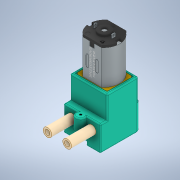
# Autodesk Inventor part: MPP20-E20
Saved by Autodesk Inventor 2020.4 (Build 244396010, 396A)
## iProperties
Created: 2021-10-01
Part Number: MPP20-E20
Material: Generic
Document SubType Name: Modeling
Designer: jonathanlim
Density: 1 g/cm^3
Appearance: Default
Author: jonathanlim
Autodesk Inventor part; units mm, degrees
ref_plane "YZ Plane" through (0, 0, 0) normal (1, 0, 0) x (0, 1, 0)
ref_plane "XZ Plane" through (0, 0, 0) normal (0, 1, 0) x (-1, 0, 0)
ref_plane "XY Plane" through (0, 0, 0) normal (0, 0, 1) x (1, 0, 0)
sketch "Sketch1" plane through (0, 0, 0) normal (0, 1, 0) x (-1, 0, 0)
  line L0 (-7.5, 8.3) -> (7.5, 8.3)
  line L1 (7.5, 8.3) -> (7.5, -8.3)
  line L2 (7.5, -8.3) -> (-7.5, -8.3)
  line L3 (-7.5, -8.3) -> (-7.5, 8.3)
  line L4 (-7.5, 8.3) -> (7.5, -8.3) construction
  line L5 (7.5, 8.3) -> (-7.5, -8.3) construction
  point P0 (0, 0)
  dimension "d0" = 15
  dimension "d1" = 16.6
  constraints: 12 end point, 2 midpoint, 2 parallel, 1 horizontal, 1 perpendicular
  measures "d0" distance of L1.end L2.end
  measures "d1" distance of L0.end L1.end
extrude "Extrusion1" add sketch "Sketch1" along normal blind 10.35
sketch "Sketch2" plane through (0, 10.35, 0) normal (0, 1, 0) x (1, 0, 0)
  line L0 (-7.5, -5.55) -> (7.5, -5.55)
  line L1 (7.5, -5.55) -> (7.5, 7.25)
  line L2 (7.5, 7.25) -> (-7.5, 7.25)
  line L3 (-7.5, 7.25) -> (-7.5, -5.55)
  line L4 (-7.5, -5.55) -> (7.5, 7.25) construction
  line L5 (7.5, -5.55) -> (-7.5, 7.25) construction
  line L6 (-7.5, -8.3) -> (7.5, -8.3) projected
  point P0 (0, 0)
  point P1 (0, 0.85)
  point P2 (0, 0.85)
  dimension "d4" = 12.8
  dimension "d5" = 2.75
  constraints: 12 end point, 3 midpoint, 2 parallel, 1 horizontal, 1 perpendicular, 1 vertical alignment
  measures "d4" distance of L1.end L0.end
  measures "d5" distance between parallel lines of L6 L0
extrude "Extrusion2" add sketch "Sketch2" along normal blind 9.2
sketch "Sketch3" plane through (0, 19.55, 0) normal (0, 1, 0) x (1, 0, 0)
  line L0 (-3.8, -4.15) -> (3.8, -4.15)
  line L1 (3.8, -4.15) -> (3.8, 5.85)
  line L2 (3.8, 5.85) -> (-3.8, 5.85)
  line L3 (-3.8, 5.85) -> (-3.8, -4.15)
  line L4 (-3.8, -4.15) -> (3.8, 5.85) construction
  line L5 (3.8, -4.15) -> (-3.8, 5.85) construction
  line L6 (-7.5, 7.25) -> (-7.5, -5.55)
  line L7 (7.5, 7.25) -> (-7.5, 7.25)
  arc A0 (-3.8, 5.85) -> (-3.8, -4.15) centre (0.353312, 0.85) ccw
  arc A1 (3.8, -4.15) -> (3.8, 5.85) centre (-0.353312, 0.85) ccw
  point P0 (0, 0.85)
  dimension "d10" = 7.6
  dimension "d11" = 10
  dimension "d12" = 7.5
  dimension "d13" = 1.4
  dimension "d14" = 6.5
  constraints: 12 end point, 4 point on circle, 2 centre point, 2 midpoint, 2 parallel, 1 equal radius, 1 horizontal, 1 perpendicular
  measures "d10" distance of L2.end L1.end
  measures "d11" distance of L1.end L0.end
  measures "d12" distance from line of L6 point (0, 0.85)
  measures "d13" distance between parallel lines of L7 L2
  measures "d14" radius of A0
extrude "Extrusion3" add sketch "Sketch3" along normal blind 14 separate body
sketch "Sketch6" plane through (0, 10.35, 0) normal (0, 1, 0) x (1, 0, 0)
  arc A0 (-1.910661, -8.3) -> (1.910661, -8.3) centre (0, -8.8) ccw
  line L0 (-7.5, -8.3) -> (7.5, -8.3)
  line L1 (-7.5, -8.3) -> (7.5, -8.3)
  line L2 (-1.910661, -8.3) -> (1.910661, -8.3)
  point P0 (0, 0)
  point P1 (1.910661, -8.3)
  point P2 (-1.910661, -8.3)
  dimension "d24" = 3.95
  dimension "d25" = 0.5
  constraints: 2 end point, 2 point on circle, 2 point on line, 1 centre point
  measures "d24" diameter of A0
  measures "d25" distance from line of L0 A0.centre
extrude "Extrusion6" add sketch "Sketch6" against normal blind 5.55 bodies 1
sketch "Sketch7" plane through (0, 0, 0) normal (0, -1, 0) x (1, 0, 0)
  circle A0 centre (0, 8.8) radius 1.975
  line L0 (-7.5, 8.3) -> (7.5, 8.3) projected
  point P0 (0, 0)
  dimension "d28" = 3.95
  dimension "d29" = 0.5
  constraints: 1 centre point
  measures "d28" diameter of A0
  measures "d29" distance from line of L0 A0.centre
extrude "Extrusion7" cut sketch "Sketch7" against normal up to surface (4.8 mm away) bodies 1
sketch "Sketch8" plane through (7.5, 0, 8.3) normal (0, 0, 1) x (1, 0, 0)
  circle A0 centre (-3.5, 6.85) radius 1.75
  circle A1 centre (-11.5, 6.85) radius 1.75
  line L0 (0, 0) -> (0, 10.35)
  line L1 (-5.589339, 10.35) -> (0, 10.35)
  point P0 (-7.5, 0)
  dimension "d32" = 3.5
  dimension "d33" = 8
  dimension "d34" = 3.5
  dimension "d37" = 3.5
  constraints: 2 centre point, 1 equal radius, 1 horizontal alignment
  measures "d32" diameter of A0
  measures "d33" distance of A0.centre A1.centre
  measures "d34" distance from line of L0 A0.centre
  measures "d37" distance from line of L1 A0.centre
extrude "Extrusion8" add sketch "Sketch8" along normal blind 10 separate body
sketch "Sketch12" plane through (0, 19.55, 0) normal (0, 1, 0) x (1, 0, 0)
  line L0 (-5.35, -4.4) -> (5.35, -4.4)
  line L1 (6.35, -3.4) -> (6.35, 5.1)
  line L2 (5.35, 6.1) -> (-5.35, 6.1)
  line L3 (-6.35, 5.1) -> (-6.35, -3.4)
  line L4 (-6.35, -4.4) -> (6.35, 6.1) construction
  line L5 (6.35, -4.4) -> (-6.35, 6.1) construction
  line L6 (7.5, -5.55) -> (7.5, 7.25) projected
  line L7 (7.5, 7.25) -> (-7.5, 7.25) projected
  line L8 (-7.5, -5.55) -> (7.5, -5.55) projected
  line L9 (-7.5, 7.25) -> (-7.5, -5.55) projected
  arc A0 (-5.35, 6.1) -> (-6.35, 5.1) centre (-5.35, 5.1) ccw
  arc A1 (6.35, 5.1) -> (5.35, 6.1) centre (5.35, 5.1) ccw
  arc A2 (5.35, -4.4) -> (6.35, -3.4) centre (5.35, -3.4) ccw
  arc A3 (-6.35, -3.4) -> (-5.35, -4.4) centre (-5.35, -3.4) ccw
  line L10 (-6.5, -4.55) -> (6.5, -4.55)
  line L11 (6.5, -4.55) -> (6.5, 6.25)
  line L12 (6.5, 6.25) -> (-6.5, 6.25)
  line L13 (-6.5, 6.25) -> (-6.5, -4.55)
  line L14 (-6.5, -4.55) -> (6.5, 6.25) construction
  line L15 (6.5, -4.55) -> (-6.5, 6.25) construction
  point P0 (0, 0)
  point P1 (0, 0.85)
  dimension "d52" = 1.15
  dimension "d53" = 1.15
  dimension "d54" = 1.15
  dimension "d55" = 1.15
  dimension "d56" = 1
  dimension "d57" = 1
  dimension "d58" = 1
  constraints: 24 end point, 8 point on circle, 8 point on line, 8 tangent, 4 centre point, 4 midpoint, 4 parallel, 3 equal radius, 2 horizontal, 2 perpendicular
  measures "d52" distance between parallel lines of L6 L1
  measures "d53" distance between parallel lines of L7 L2
  measures "d54" distance between parallel lines of L8 L0
  measures "d55" distance between parallel lines of L3 L9
  measures "d56" radius of A0
  measures "d57" distance between parallel lines of L7 L12
  measures "d58" distance between parallel lines of L6 L11
extrude "Extrusion11" cut sketch "Sketch12" against normal blind 1 contours L13 L12 L11 L10 bodies 1
sketch "Sketch13" plane through (0, 33.55, 0) normal (0, 1, 0) x (1, 0, 0)
  line L0 (3.8, 5.85) -> (-3.8, 5.85)
  line L1 (-3.8, 5.85) -> (3.8, 5.85)
  arc A0 (3.8, -4.15) -> (3.8, 5.85) centre (-0.353312, 0.85) ccw
  arc A1 (3.8, -4.15) -> (3.8, 5.85) centre (-0.353312, 0.85) ccw
  line L2 (-3.8, -4.15) -> (3.8, -4.15)
  arc A2 (-3.8, 5.85) -> (-3.8, -4.15) centre (0.353312, 0.85) ccw
  line L3 (-3.8, -4.15) -> (3.8, -4.15)
  line L4 (-5.35, -4.4) -> (5.35, -4.4)
  point P0 (0, 0)
  constraints: 4 end point, 4 point on circle, 2 centre point, 1 collinear, 1 parallel
extrude "Extrusion12" add sketch "Sketch13" along normal blind 1 separate body
sketch "Sketch15" plane through (0, 34.55, 0) normal (0, 1, 0) x (1, 0, 0)
  line L0 (3.5, 1.6) -> (3.8, 1.6)
  line L1 (3.8, 1.6) -> (3.8, 0.1)
  line L2 (3.8, 0.1) -> (3.5, 0.1)
  line L3 (3.5, 0.1) -> (3.5, 1.6)
  line L4 (3.5, 1.6) -> (3.8, 0.1) construction
  line L5 (3.8, 1.6) -> (3.5, 0.1) construction
  line L6 (-3.8, 1.6) -> (-3.5, 1.6)
  line L7 (-3.5, 1.6) -> (-3.5, 0.1)
  line L8 (-3.5, 0.1) -> (-3.8, 0.1)
  line L9 (-3.8, 0.1) -> (-3.8, 1.6)
  line L10 (-3.8, 1.6) -> (-3.5, 0.1) construction
  line L11 (-3.5, 1.6) -> (-3.8, 0.1) construction
  line L12 (-3.8, -4.15) -> (3.8, -4.15) projected
  point P0 (0, 0)
  point P1 (3.65, 0.85)
  point P2 (-3.65, 0.85)
  point P3 (-3.65, 0.85)
  point P4 (3.65, 0.85)
  dimension "d67" = 0.3
  dimension "d68" = 1.5
  dimension "d69" = 5
  dimension "d70" = 7.6
  dimension "d71" = 3.65
  constraints: 24 end point, 6 midpoint, 4 parallel, 2 equal length, 2 horizontal, 2 perpendicular, 1 horizontal alignment
  measures "d67" distance of L1.end L2.end
  measures "d68" distance of L0.end L1.end
  measures "d69" distance from line of L12 point (-3.65, 0.85)
  measures "d70" distance between parallel lines of L1 L9
  measures "d71" horizontal distance of point (0, 0) point (-3.65, 0.85)
extrude "Extrusion14" add sketch "Sketch15" along normal blind 1.5 separate body
sketch "Sketch16" plane through (3.8, 34.55, -0.1) normal (1, 0, 0) x (0, 0, -1)
  line L0 (1.5, 0) -> (1.5, 1.5)
  line L1 (0, 0) -> (0, 1.5)
  arc A0 (1.5, 1.299038) -> (0, 1.299038) centre (0.75, 0) ccw
  line L2 (0, 1.5) -> (1.5, 1.5)
  line L3 (0, 1.299038) -> (0, 1.5)
  line L4 (0, 1.5) -> (1.5, 1.5)
  line L5 (1.5, 1.5) -> (1.5, 1.299038)
  line L6 (1.5, 1.5) -> (0, 1.5)
  circle A1 centre (0.75, 0.85) radius 0.375
  point P0 (-0.1, -34.55)
  point P1 (0.75, 1.5)
  dimension "d74" = 1.5
  dimension "d75" = 1.5
  dimension "d78" = 0.75
  dimension "d79" = 0.65
  constraints: 6 end point, 2 centre point, 2 collinear, 2 point on circle, 2 point on line, 1 horizontal alignment, 1 perpendicular
  measures "d74" radius of A0
  measures "d75" distance from line of L2 A0.centre
  measures "d78" diameter of A1
  measures "d79" distance from line of L2 A1.centre
extrude "Extrusion15" cut sketch "Sketch16" against normal through all bodies 5
sketch "Sketch17" plane through (0, 34.55, 0) normal (0, 1, 0) x (1, 0, 0)
  circle A0 centre (0, 0.85) radius 2.5
  point P0 (0, 0)
  dimension "d80" = 5
  dimension "d81" = 0.85
  constraints: 1 centre point
  measures "d80" diameter of A0
  measures "d81" distance of A0.centre point (0, 0)
extrude "Extrusion16" add sketch "Sketch17" along normal blind 1 bodies 4
sketch "Sketch18" plane through (0, 35.55, -0.85) normal (0, 1, 0) x (1, 0, 0)
  circle A0 centre (0, 0) radius 1
  circle A1 centre (0, 0) radius 2.5 projected
  point P0 (0, -0.85)
  dimension "d84" = 1.5
  constraints: 1 centre point, 1 coincident
  measures "d84" radial gap between concentric circles of A1 A0
extrude "Extrusion17" cut sketch "Sketch18" against normal blind 0.5 contours A0 bodies 4
fillet "Fillet3" radius 2 2 edges at (7.5, 5.175, -8.3) (-7.5, 5.175, -8.3)
fillet "Fillet4" radius 0.5 28 edges at (7.5, 14.95, 5.55) (7.26, 14.95, -7.25) (-7.26, 14.95, -7.25) (-7.5, 14.95, 5.55) (6.9142, 0, -7.7142) (0, 0, -8.3) (-6.9142, 0, -7.7142) (-7.5, 0, 1) (7.5, 0, 1) (-7.5, 5.175, 8.3) (-4.7053, 0, 8.3) (0, 0, 6.825) (4.7053, 0, 8.3) (7.5, 5.175, 8.3) (1.9107, 2.4, 8.3) (-1.9107, 2.4, 8.3) (0, 4.8, 10.775) (0, 10.35, 10.775) (7.5, 10.35, 6.925) (4.7053, 10.35, 8.3) (-4.7053, 10.35, 8.3) (-7.5, 10.35, 6.925) (7.4391, 19.55, -6.7899) (7.5, 19.55, -0.375) (0, 19.55, 5.55) (-7.4391, 19.55, -6.7899) (-7.5, 19.55, -0.375) (0, 19.55, -7.25)
sketch "Sketch19" plane through (0, 4.8, 0) normal (0, -1, 0) x (1, 0, 0)
  circle A0 centre (0, 8.8) radius 1.225
  arc A1 (1.387669, 8.3) -> (-1.387669, 8.3) centre (0, 8.8) ccw
  point P0 (0, 0)
  dimension "d91" = 2.45
  constraints: 1 centre point, 1 concentric
  measures "d91" diameter of A0
extrude "Extrusion18" add sketch "Sketch19" along normal blind 0.5 separate body
sketch "Sketch20" plane through (0, 0, 0) normal (0, -1, 0) x (1, 0, 0)
  circle A0 centre (0, -0.85) radius 3.35
  circle A1 centre (0, -0.85) radius 2.5 projected
  point P0 (0, 0)
  dimension "d94" = 6.7
  constraints: 1 centre point, 1 concentric
  measures "d94" diameter of A0
extrude "Extrusion19" add sketch "Sketch20" along normal blind 1.75 contours A0 | A1 bodies 1
fillet "Fillet5" radius 0.5 1 edges at (-3.35, -1.75, -0.85)
sketch "Sketch21" plane through (0, 0, 0) normal (0, -1, 0) x (1, 0, 0)
  circle A0 centre (-5.5, -6.3) radius 1.225
  circle A1 centre (5.5, -6.3) radius 1.225
  arc A2 (-7, -6.3) -> (-5.5, -7.8) centre (-5.5, -6.3) ccw projected
  arc A3 (5.5, -7.8) -> (7, -6.3) centre (5.5, -6.3) ccw projected
  point P0 (0, 0)
  dimension "d98" = 2.45
  constraints: 2 centre point, 2 concentric, 1 equal radius
  measures "d98" diameter of A0
extrude "Extrusion20" add sketch "Sketch21" along normal blind 0.5 separate body
fillet "Fillet6" radius 0.25 3 edges at (-1.225, 4.3, 8.8) (-6.725, -0.5, -6.3) (4.275, -0.5, -6.3)
sketch "Sketch22" plane through (0, -1.75, -0.85) normal (0, -1, 0) x (1, 0, 0)
  circle A0 centre (0, 1.25) radius 0.5
  circle A1 centre (0, -1.25) radius 0.5
  circle A2 centre (0, 0) radius 1 projected
  point P0 (0, 0.85)
  dimension "d102" = 1
  dimension "d103" = 1
  dimension "d104" = 1.25
  dimension "d105" = 1.25
  constraints: 2 centre point
  measures "d102" diameter of A0
  measures "d103" diameter of A1
  measures "d104" distance of A0.centre A2.centre
  measures "d105" distance of A1.centre A2.centre
extrude "Extrusion21" cut sketch "Sketch22" against normal blind 1 contours A0 A2 | A2 A0 | A2 A1 | A1 A2 bodies 1
sketch "Sketch23" plane through (-5.5, -0.5, -6.3) normal (0, -1, 0) x (1, 0, 0)
  line L0 (-2, 14.1) -> (-2, 0)
  line L1 (10.593414, -0.654074) -> (11.654074, 0.406586)
  line L2 (11.654074, 0.406586) -> (11.406586, 0.654074)
  line L3 (11.406586, 0.654074) -> (10.345926, -0.406586)
  line L4 (10.345926, -0.406586) -> (10.593414, -0.654074)
  line L5 (10.593414, -0.654074) -> (11.406586, 0.654074) construction
  line L6 (11.654074, 0.406586) -> (10.345926, -0.406586) construction
  line L7 (10.593414, -0.654074) -> (12.093414, -0.654074) construction
  circle A0 centre (11, 0) radius 1.225
  line L8 (11.654074, -0.406586) -> (10.593414, 0.654074)
  line L9 (10.593414, 0.654074) -> (10.345926, 0.406586)
  line L10 (10.345926, 0.406586) -> (11.406586, -0.654074)
  line L11 (11.406586, -0.654074) -> (11.654074, -0.406586)
  line L12 (11.654074, -0.406586) -> (10.345926, 0.406586) construction
  line L13 (10.593414, 0.654074) -> (11.406586, -0.654074) construction
  line L14 (11.654074, -0.406586) -> (13.154074, -0.406586) construction
  line L15 (-0.654074, -0.406586) -> (0.406586, 0.654074)
  line L16 (0.406586, 0.654074) -> (0.654074, 0.406586)
  line L17 (0.654074, 0.406586) -> (-0.406586, -0.654074)
  line L18 (-0.406586, -0.654074) -> (-0.654074, -0.406586)
  line L19 (-0.654074, -0.406586) -> (0.654074, 0.406586) construction
  line L20 (0.406586, 0.654074) -> (-0.406586, -0.654074) construction
  line L21 (-0.654074, -0.406586) -> (0.845926, -0.406586) construction
  line L22 (0.406586, -0.654074) -> (-0.654074, 0.406586)
  line L23 (-0.654074, 0.406586) -> (-0.406586, 0.654074)
  line L24 (-0.406586, 0.654074) -> (0.654074, -0.406586)
  line L25 (0.654074, -0.406586) -> (0.406586, -0.654074)
  line L26 (0.406586, -0.654074) -> (-0.406586, 0.654074) construction
  line L27 (-0.654074, 0.406586) -> (0.654074, -0.406586) construction
  line L28 (0.406586, -0.654074) -> (1.906586, -0.654074) construction
  circle A1 centre (0, 0) radius 1.225
  point P0 (5.5, 6.3)
  point P1 (0, 0)
  point P2 (0, 0)
  point P3 (10.752513, 0)
  point P4 (11, -0.247487)
  point P5 (11.247487, 0)
  point P6 (11, 0.247487)
  point P7 (-0.247487, 0)
  point P8 (0, -0.247487)
  point P9 (0.247487, 0)
  point P10 (0, 0.247487)
  dimension "d122" = 1.5
  dimension "d123" = 45
  dimension "d124" = 0.35
  dimension "d125" = 0
  dimension "d126" = 0
  dimension "d127" = 1.5
  dimension "d128" = 135
  dimension "d129" = 0.35
  dimension "d130" = 1.5
  dimension "d131" = 45
  dimension "d132" = 0.35
  dimension "d133" = 1.5
  dimension "d134" = 135
  dimension "d135" = 0.35
  dimension "d136" = 0
  dimension "d137" = 0
  constraints: 56 end point, 9 midpoint, 9 parallel, 4 equal length, 4 horizontal, 4 perpendicular
  measures "d122" distance of L1.start L1.end
  measures "d123" angle of L7 L1
  measures "d124" distance of L2.end L1.end
  measures "d125" distance of A0.centre point (11, 0)
  measures "d126" distance of A0.centre point (11, 0)
  measures "d127" distance of L8.start L8.end
  measures "d128" angle of L14 L8
  measures "d129" distance of L9.end L8.end
  measures "d130" distance of L15.start L15.end
  measures "d131" angle of L21 L15
  measures "d132" distance of L15.end L16.end
  measures "d133" distance of L22.start L22.end
  measures "d134" angle of L28 L22
  measures "d135" distance of L22.end L23.end
  measures "d136" distance of A1.centre point (0, 0)
  measures "d137" distance of A1.centre point (0, 0)
extrude "Extrusion22" cut sketch "Sketch23" against normal blind 0.25 contours L4 L3 L10 L1 | L10 L3 L8 L1 | L1 L8 L11 L10 | L8 L3 L2 L1 | L10 L9 L8 L3 | L15 L22 L17 L18 | L22 L23 L24 L15 | L15 L24 L17 L22 | L15 L16 L17 L24 | L17 L24 L25 L22 bodies 7
sketch "Sketch24" plane through (0, 4.3, 8.8) normal (0, -1, 0) x (1, 0, 0)
  line L0 (-0.406586, -0.654074) -> (0.654074, 0.406586)
  line L1 (0.654074, 0.406586) -> (0.406586, 0.654074)
  line L2 (0.406586, 0.654074) -> (-0.654074, -0.406586)
  line L3 (-0.654074, -0.406586) -> (-0.406586, -0.654074)
  line L4 (-0.406586, -0.654074) -> (0.406586, 0.654074) construction
  line L5 (0.654074, 0.406586) -> (-0.654074, -0.406586) construction
  line L6 (-0.406586, -0.654074) -> (1.093414, -0.654074) construction
  line L7 (0.406586, -0.654074) -> (-0.654074, 0.406586)
  line L8 (-0.654074, 0.406586) -> (-0.406586, 0.654074)
  line L9 (-0.406586, 0.654074) -> (0.654074, -0.406586)
  line L10 (0.654074, -0.406586) -> (0.406586, -0.654074)
  line L11 (0.406586, -0.654074) -> (-0.406586, 0.654074) construction
  line L12 (-0.654074, 0.406586) -> (0.654074, -0.406586) construction
  line L13 (0.406586, -0.654074) -> (1.906586, -0.654074) construction
  circle A0 centre (0, 0) radius 1.225
  point P0 (0, -8.8)
  point P1 (0, 0)
  point P2 (0.247487, 0)
  point P3 (0, 0.247487)
  point P4 (-0.247487, 0)
  point P5 (0, -0.247487)
  dimension "d140" = 1.5
  dimension "d141" = 45
  dimension "d142" = 0.35
  dimension "d143" = 1.5
  dimension "d144" = 135
  dimension "d145" = 0.35
  dimension "d146" = 0
  dimension "d147" = 0
  constraints: 28 end point, 5 midpoint, 5 parallel, 2 equal length, 2 horizontal, 2 perpendicular
  measures "d140" distance of L0.start L0.end
  measures "d141" angle of L6 L0
  measures "d142" distance of L1.end L0.end
  measures "d143" distance of L7.start L7.end
  measures "d144" angle of L13 L7
  measures "d145" distance of L7.end L8.end
  measures "d146" distance of point (0, 0) A0.centre
  measures "d147" distance of A0.centre point (0, 0)
extrude "Extrusion23" cut sketch "Sketch24" against normal blind 0.25 contours L3 L2 L7 L0 | L7 L2 L9 L0 | L0 L9 L10 L7 | L9 L2 L1 L0 | L7 L8 L9 L2 bodies 6
sketch "Sketch25" plane through (0, 10.35, 0) normal (0, 1, 0) x (1, 0, 0)
  circle A0 centre (0, -8.8) radius 0.425
  arc A1 (-1.084262, -7.8) -> (1.084262, -7.8) centre (0, -8.8) ccw
  point P0 (0, 0)
  dimension "d150" = 0.85
  constraints: 1 centre point, 1 concentric
  measures "d150" diameter of A0
extrude "Extrusion24" cut sketch "Sketch25" against normal blind 0.5 bodies 1
sketch "Sketch26" plane through (-3.8, 19.55, 4.15) normal (0, 0, 1) x (1, 0, 0)
  line L0 (1.875, 4.15) -> (1.875, 8.9) construction
  line L1 (2.45, 4.725) -> (2.45, 8.325)
  line L2 (1.3, 8.325) -> (1.3, 4.725)
  arc A0 (1.3, 4.725) -> (2.45, 4.725) centre (1.875, 4.725) ccw
  arc A1 (2.45, 8.325) -> (1.3, 8.325) centre (1.875, 8.325) ccw
  line L3 (5.725, 4.15) -> (5.725, 8.9) construction
  line L4 (6.3, 4.725) -> (6.3, 8.325)
  line L5 (5.15, 8.325) -> (5.15, 4.725)
  arc A2 (5.15, 4.725) -> (6.3, 4.725) centre (5.725, 4.725) ccw
  arc A3 (6.3, 8.325) -> (5.15, 8.325) centre (5.725, 8.325) ccw
  line L6 (0, 0) -> (0, 14) projected
  line L7 (0, 15) -> (7.6, 15) projected
  point P0 (3.8, -19.55)
  point P1 (1.875, 6.525)
  point P2 (5.725, 6.525)
  dimension "d153" = 4.75
  dimension "d154" = 1.15
  dimension "d155" = 4.75
  dimension "d156" = 1.15
  dimension "d157" = 5
  dimension "d158" = 1.3
  dimension "d159" = 6.1
  constraints: 16 end point, 12 point on circle, 8 tangent, 4 centre point, 4 point on line, 2 midpoint, 2 parallel, 2 vertical, 1 horizontal alignment
  measures "d153" distance of L0.start L0.end
  measures "d154" diameter of A1
  measures "d155" distance of L3.start L3.end
  measures "d156" diameter of A3
  measures "d157" distance between parallel lines of L4 L2
  measures "d158" distance between parallel lines of L6 L2
  measures "d159" distance from line of L7 L0.end
extrude "Extrusion25" cut sketch "Sketch26" against normal blind 0.05 bodies 2
sketch "Sketch27" plane through (3.8, 19.55, -5.85) normal (0, 0, -1) x (-1, 0, 0)
  arc A0 (1.3, 4.725) -> (2.45, 4.725) centre (1.875, 4.725) ccw projected
  arc A1 (2.45, 8.325) -> (1.3, 8.325) centre (1.875, 8.325) ccw projected
  line L0 (1.875, 4.725) -> (1.875, 8.325) construction
  line L1 (2.45, 4.725) -> (2.45, 8.325)
  line L2 (1.3, 8.325) -> (1.3, 4.725)
  arc A2 (1.3, 4.725) -> (2.45, 4.725) centre (1.875, 4.725) ccw
  arc A3 (2.45, 8.325) -> (1.3, 8.325) centre (1.875, 8.325) ccw
  line L3 (5.15, 8.325) -> (5.15, 4.725) projected
  line L4 (5.15, 4.725) -> (5.15, 8.325) construction
  line L5 (5.725, 4.725) -> (5.725, 8.325)
  line L6 (4.575, 8.325) -> (4.575, 4.725)
  arc A4 (4.575, 4.725) -> (5.725, 4.725) centre (5.15, 4.725) ccw
  arc A5 (5.725, 8.325) -> (4.575, 8.325) centre (5.15, 8.325) ccw
  point P0 (3.8, -19.55)
  point P1 (1.875, 6.525)
  point P2 (5.15, 6.525)
  dimension "d162" = 1.15
  constraints: 16 end point, 8 point on circle, 8 tangent, 4 centre point, 3 equal length, 2 midpoint, 1 vertical
  measures "d162" diameter of A5
extrude "Extrusion26" cut sketch "Sketch27" against normal blind 0.15 bodies 2
sketch "Sketch28" plane through (0, 34.55, 0) normal (0, 1, 0) x (1, 0, 0)
  arc A0 (-3.8, 5.85) -> (-3.8, -4.15) centre (0.353312, 0.85) ccw
  arc A1 (-6.07689, 1.8) -> (-6.07689, -0.1) centre (0.353312, 0.85) ccw
  line L0 (-6.07689, 1.8) -> (-6.07689, -0.1) construction
  line L1 (-6.07689, 1.8) -> (-4.17689, 1.8) construction
  line L2 (-6.07689, 1.8) -> (-4.92689, 1.8)
  line L3 (-4.92689, 1.8) -> (-4.92689, -0.1)
  line L4 (-4.92689, -0.1) -> (-6.07689, -0.1)
  line L5 (-6.07689, -0.1) -> (-6.07689, 1.8)
  line L6 (3.8, 5.85) -> (-3.8, 5.85) construction
  line L7 (0, 5.85) -> (0, -4.15) construction
  arc A2 (6.07689, -0.1) -> (6.07689, 1.8) centre (-0.353312, 0.85) ccw
  line L8 (6.07689, 1.8) -> (6.07689, -0.1) construction
  line L9 (6.07689, 1.8) -> (4.17689, 1.8) construction
  line L10 (6.07689, 1.8) -> (4.92689, 1.8)
  line L11 (4.92689, 1.8) -> (4.92689, -0.1)
  line L12 (4.92689, -0.1) -> (6.07689, -0.1)
  line L13 (6.07689, -0.1) -> (6.07689, 1.8)
  point P0 (0, 0)
  point P1 (-6.07689, -0.1)
  point P2 (6.07689, -0.1)
  dimension "d165" = 90
  dimension "d166" = 1.9
  dimension "d167" = 1.15
  constraints: 26 end point, 7 symmetric about line, 6 point on circle, 2 centre point, 2 horizontal, 2 parallel, 2 perpendicular, 1 midpoint, 1 vertical, 1 other
  measures "d165" angle of L0 L1
  measures "d166" distance of L0.start L0.end
  measures "d167" distance of L3.end L4.end
extrude "Extrusion27" cut sketch "Sketch28" against normal blind 2.45 bodies 4
sketch "Sketch29" plane through (-3.8, 19.55, 4.15) normal (0, 0, 1) x (1, 0, 0)
  line L0 (0, 14) -> (7.6, 14) projected
  line L1 (2.925, 14) -> (4.675, 14)
  line L2 (4.675, 14) -> (4.675, 12.25)
  line L3 (4.675, 12.25) -> (2.925, 12.25)
  line L4 (2.925, 12.25) -> (2.925, 14)
  line L5 (0, 0) -> (0, 14) projected
  point P0 (3.8, -19.55)
  dimension "d170" = 1.75
  dimension "d171" = 1.75
  dimension "d172" = 2.925
  constraints: 8 end point, 2 parallel, 1 horizontal, 1 perpendicular, 1 point on line
  measures "d170" distance of L2.end L3.end
  measures "d171" distance of L1.end L2.end
  measures "d172" distance between parallel lines of L5 L4
extrude "Extrusion28" cut sketch "Sketch29" against normal blind 0.15 bodies 2
sketch "Sketch30" plane through (0, 34.55, 0) normal (0, 1, 0) x (1, 0, 0)
  circle A0 centre (-3, -2.9) radius 0.825
  circle A1 centre (0, 4.6) radius 0.825
  line L0 (3.8, 5.85) -> (-3.8, 5.85) projected
  line L1 (-3.8, -4.15) -> (3.8, -4.15) projected
  point P0 (0, 0)
  dimension "d176" = 1.25
  dimension "d180" = 1.65
  dimension "d181" = 0.8
  dimension "d182" = 1.25
  constraints: 2 centre point, 1 equal radius
  measures "d176" distance from line of L0 A1.centre
  measures "d180" diameter of A0
  measures "d181" horizontal distance of L1.start A0.centre
  measures "d182" distance from line of L1 A0.centre
extrude "Extrusion29" cut sketch "Sketch30" against normal blind 0.15 bodies 4
sketch "Sketch31" plane through (0, 34.55, 0) normal (0, 1, 0) x (1, 0, 0)
  circle A0 centre (3, -2.9) radius 0.825
  arc A1 (3.8, -4.15) -> (3.8, 5.85) centre (-0.353312, 0.85) ccw
  line L0 (-3.8, -4.15) -> (3.8, -4.15)
  point P0 (0, 0)
  dimension "d185" = 1.65
  dimension "d186" = 0.8
  dimension "d187" = 1.25
  constraints: 1 centre point
  measures "d185" diameter of A0
  measures "d186" horizontal distance of A0.centre L0.end
  measures "d187" distance from line of L0 A0.centre
extrude "Extrusion30" cut sketch "Sketch31" against normal blind 0.35 bodies 4
sketch "Sketch32" plane through (3, 34.2, 2.9) normal (0, 1, 0) x (1, 0, 0)
  circle A0 centre (0, 0) radius 0.825
  arc A1 (-0.681314, -0.465228) -> (0.689192, -0.465228) centre (0.003939, 0.00726) ccw
  line L0 (0.689192, -0.465228) -> (-0.681314, -0.465228) construction
  line L1 (0.689192, -0.465228) -> (2.059698, -0.465228) construction
  line L2 (1.003939, 0.10726) -> (-0.996061, 0.10726)
  line L3 (-0.996061, 0.10726) -> (-0.996061, -0.09274)
  line L4 (-0.996061, -0.09274) -> (1.003939, -0.09274)
  line L5 (1.003939, -0.09274) -> (1.003939, 0.10726)
  line L6 (1.003939, 0.10726) -> (-0.996061, -0.09274) construction
  line L7 (-0.996061, 0.10726) -> (1.003939, -0.09274) construction
  line L8 (0.103939, 1.00726) -> (-0.096061, 1.00726)
  line L9 (-0.096061, 1.00726) -> (-0.096061, -0.99274)
  line L10 (-0.096061, -0.99274) -> (0.103939, -0.99274)
  line L11 (0.103939, -0.99274) -> (0.103939, 1.00726)
  line L12 (0.103939, 1.00726) -> (-0.096061, -0.99274) construction
  line L13 (-0.096061, 1.00726) -> (0.103939, -0.99274) construction
  point P0 (-3, 2.9)
  point P1 (0.103939, -0.09274)
  point P2 (0.103939, 0.10726)
  point P3 (-0.096061, 0.10726)
  point P4 (-0.096061, -0.09274)
  dimension "d190" = 180
  dimension "d191" = 2
  dimension "d192" = 0.2
  dimension "d193" = 0.2
  dimension "d194" = 2
  constraints: 28 end point, 4 midpoint, 4 parallel, 3 horizontal, 2 perpendicular, 2 point on circle, 1 centre point, 1 collinear, 2 other
  measures "d190" angle of L0 L1
  measures "d191" distance of L4.end L3.end
  measures "d192" distance of L3.end L2.end
  measures "d193" distance of L10.end L9.end
  measures "d194" distance of L9.end L8.end
extrude "Extrusion31" add sketch "Sketch32" along normal blind 0.25 contours A0 L4 L11 L2 | A0 L2 L5 L4 | L11 L2 L9 A0 | A0 L9 L8 L11 | L11 L4 L9 L2 | L11 L10 L9 A0 | A0 L9 L4 L11 | L9 L4 A0 L2 | A0 L4 L3 L2 bodies 4
sketch "Sketch33" plane through (-3.8, 19.55, 4.15) normal (0, 0, 1) x (1, 0, 0)
  line L0 (2.642909, -6.412403) -> (2.642909, 19.83399) construction
  line L1 (2.642909, 19.83399) -> (10.827922, 19.83399) construction
  line L2 (10.827922, 19.83399) -> (10.827922, -6.412403) construction
  line L3 (10.827922, -6.412403) -> (2.642909, -6.412403) construction
  point P0 (3.8, -19.55)
  constraints: 2 other
sketch "Sketch34" plane through (4, 6.85, 18.3) normal (0, 0, 1) x (1, 0, 0)
  circle A0 centre (0, 0) radius 1
  circle A1 centre (0, 0) radius 1.75 projected
  circle A2 centre (-8, 0) radius 1
  circle A3 centre (-8, 0) radius 1.75 projected
  point P0 (-4, -6.85)
  dimension "d198" = 0.75
  constraints: 2 centre point, 2 coincident, 1 concentric, 1 equal radius
  measures "d198" radial gap between concentric circles of A1 A0
extrude "Extrusion32" cut sketch "Sketch34" against normal blind 10 contours A0 | A2 bodies 3
body "Solid1"
body "Solid2"
body "Solid3"
body "Solid4"
body "Solid5"
body "Solid6"
body "Solid7"
